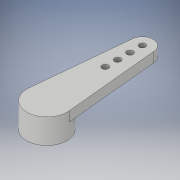
# Autodesk Inventor part: ServoHorn
Saved by Autodesk Inventor 2018 (Build 220112000, 112)
## iProperties
Created: 2019-06-13
Part Number: ServoHorn
Material: Generic
Document SubType Name: Modeling
Designer: anirudh
Density: 1 g/cm^3
Appearance: Default
Author: anirudh
Autodesk Inventor part; units mm, degrees
ref_plane "YZ Plane" through (0, 0, 0) normal (1, 0, 0) x (0, 1, 0)
ref_plane "XZ Plane" through (0, 0, 0) normal (0, 1, 0) x (-1, 0, 0)
ref_plane "XY Plane" through (0, 0, 0) normal (0, 0, 1) x (1, 0, 0)
sketch "Sketch1" plane through (0, 0, 0) normal (0, 1, 0) x (-1, 0, 0)
  circle A0 centre (0, 0) radius 4.1275
  dimension "d0" = 8.255
  constraints: 1 centre point, 1 coincident
  measures "d0" diameter of A0
extrude "Extrusion1" add sketch "Sketch1" along normal blind 5.08
sketch "Sketch2" plane through (0, 5.08, 0) normal (0, 1, 0) x (1, 0, 0)
  circle A0 centre (0, 0) radius 4.1275 projected
  arc A1 (2.2225, 19.6215) -> (-2.2225, 19.6215) centre (0, 19.6215) ccw
  line L0 (-2.2225, 19.6215) -> (-4.1041, 0.4388)
  line L1 (4.1041, 0.4388) -> (2.2225, 19.6215)
  arc A2 (-4.1041, 0.4388) -> (4.1041, 0.4388) centre (0, 0) ccw
  dimension "d4" = 4.445
  constraints: 6 point on circle, 4 end point, 2 centre point, 1 coincident
  measures "d4" diameter of A1
extrude "Extrusion2" add sketch "Sketch2" against normal blind 2.032
sketch "Sketch3" plane through (0, 5.08, 0) normal (0, 1, 0) x (1, 0, 0)
  arc A0 (2.2225, 19.6215) -> (-2.2225, 19.6215) centre (0, 19.6215) ccw projected
  circle A1 centre (0, 19.6215) radius 0.635
  circle A2 centre (0, 17.0815) radius 0.6558
  circle A3 centre (0, 14.5415) radius 0.6558
  circle A4 centre (0, 12.0015) radius 0.6558
  point P0 (0, 0)
  dimension "d7" = 1.27
  constraints: 4 centre point, 1 coincident
  measures "d7" diameter of A1
extrude "Extrusion3" cut sketch "Sketch3" against normal blind 3.6195
body "Solid1"
